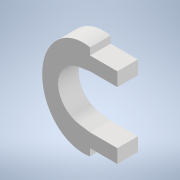
# Autodesk Inventor part: Falange proxima
Saved by Autodesk Inventor 2020 (Build 240168000, 168)
## iProperties
Created: 2021-08-19
Part Number: Falange proxima
Material: Generic
Document SubType Name: Modeling
Designer: chalo
Density: 1 g/cm^3
Appearance: Default
Author: chalo
Autodesk Inventor part; units mm, degrees
ref_plane "YZ Plane" through (0, 0, 0) normal (1, 0, 0) x (0, 1, 0)
ref_plane "XZ Plane" through (0, 0, 0) normal (0, 1, 0) x (-1, 0, 0)
ref_plane "XY Plane" through (0, 0, 0) normal (0, 0, 1) x (1, 0, 0)
sketch "Sketch1" plane through (0, 0, 0) normal (0, 0, 1) x (1, 0, 0)
  line L0 (-3, 9.0956) -> (-3, 9.6082) construction
  line L1 (-3, 9.6082) -> (3, 9.6082) construction
  ellipse E0 centre (-4.5, 3.8041) end of major axis (-4.5, -6.6959) minor radius 9 (3, 9.6082) -> (3, -2) ccw construction
  line L2 (3, -2) -> (-3, -2) construction
  line L3 (-3, -2) -> (-3, -1.4874) construction
  arc A0 (-3, 9.0956) -> (-3, -1.4874) centre (-4.5, 3.8041) ccw construction
  line L4 (3, 9.6082) -> (-3, 9.6082)
  line L5 (-3, 9.6082) -> (-3, 12.6082)
  line L6 (-3, 12.6082) -> (3, 12.6082)
  line L7 (3, 12.6082) -> (3, 9.6082)
  line L8 (-4.5, 3.8041) -> (5.5, 3.8041) construction
  line L9 (-3, -2) -> (3, -2) construction
  line L10 (-3, -2) -> (-3, -5)
  line L11 (-3, -5) -> (3, -5)
  line L12 (3, -5) -> (3, -2)
  line L13 (3, -2) -> (-3, -2)
  line L14 (-3, 9.0956) -> (-3, 9.6082) projected
  line L15 (-3, 9.6082) -> (3, 9.6082) projected
  ellipse E1 centre (-4.5, 3.8041) end of major axis (-4.5, -6.6959) minor radius 9 (3, 9.6082) -> (3, -2) ccw projected
  line L16 (3, -2) -> (-3, -2) projected
  line L17 (-3, -2) -> (-3, -1.4874) projected
  arc A1 (-3, 9.0956) -> (-3, -1.4874) centre (-4.5, 3.8041) ccw projected
  line L18 (-3, 12.6082) -> (-3, 14.1572)
  line L19 (-3, -5) -> (-3, -6.549)
  line L20 (-3, -2) -> (-5.3558, -1.6289)
  line L21 (-3, 9.6082) -> (-5.3558, 9.2371)
  point P0 (0, 0)
  dimension "d0" = 6
  dimension "d1" = 3
  dimension "d2" = 10
  constraints: 28 end point, 4 symmetric about line, 2 horizontal, 2 parallel, 2 point on circle, 2 tangent, 1 collinear, 1 perpendicular, 1 point on line, 1 vertical, 4 other
  measures "d0" distance of L5.end L6.end
  measures "d1" distance of L4.end L5.end
  measures "d2" distance of L8.start L8.end
extrude "Extrusion1" add sketch "Sketch1" along normal blind 16 and the other way blind 6.5 contours E1 L6 L7 | L4 L5 L6 E1 | L21 A1 L20 L10 L19 E1 L18 L5 | L13 E1 L11 L10 | E1 L12 L11
sketch "Sketch2" plane through (-3, 12.6082, 16) normal (0, 1, 0) x (1, 0, 0)
  circle A0 centre (3, 19.5) radius 1.6 projected
  point P0 (3, 16)
extrude "Extrusion2" cut sketch "Sketch2" against normal through all
fillet "Fillet1" radius 2 2 edges at (3, 11.1082, -6.5) (3, -3.5, -6.5)
body "Solid1"
